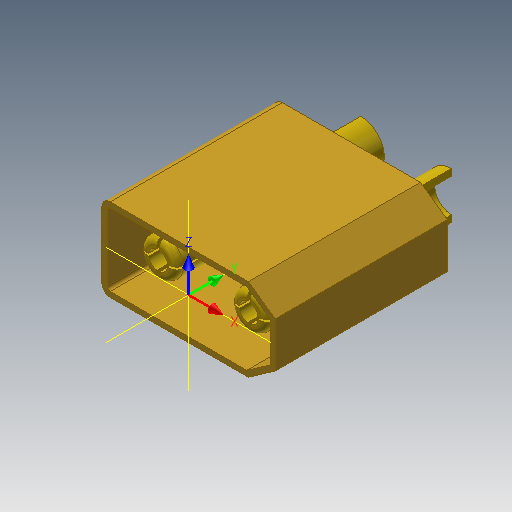
# Autodesk Inventor part: XT90 Male
Saved by Autodesk Inventor 2018 (Build 220112000, 112)
## iProperties
Created: 2021-08-31
Part Number: XT90 Male
Material: PPS-Kunststoff
Document SubType Name: Modeling
Designer: A. Gieck
Mass: 3.12149 g
Surface Area: 36.0039 cm^2
Volume: 1.90683 cm^3
Density: 1.637 g/cm^3
Appearance: Stecker Orange
RuleStatus: InUse
Author: A. Gieck
Autodesk Inventor part; units mm, degrees
ref_plane "YZ Plane" through (0, 0, 0) normal (1, 0, 0) x (0, 1, 0)
ref_plane "XZ Plane" through (0, 0, 0) normal (0, 1, 0) x (-1, 0, 0)
ref_plane "XY Plane" through (0, 0, 0) normal (0, 0, 1) x (1, 0, 0)
sketch "Skizze5" plane through (0, 0, 0) normal (0, 1, 0) x (-1, 0, 0)
  line L0 (10.475, 5) -> (-10.475, 5) construction
  line L1 (-10.475, 5) -> (-10.475, -5) construction
  line L2 (-10.475, -5) -> (10.475, -5) construction
  line L3 (10.475, -5) -> (10.475, 5) construction
  line L4 (9.475, 5) -> (-7.226, 5)
  line L5 (-7.226, 5) -> (-7.226, -5) construction
  line L6 (-7.226, -5) -> (9.475, -5)
  line L7 (10.475, -4) -> (10.475, 4)
  line L8 (-7.226, -5) -> (-10.475, -2.725)
  line L9 (-10.475, -2.725) -> (-10.475, 2.725)
  line L10 (-7.226, 5) -> (-10.475, 2.725)
  arc A0 (10.475, 4) -> (9.475, 5) centre (9.475, 4) ccw
  arc A1 (9.475, -5) -> (10.475, -4) centre (9.475, -4) ccw
  line L11 (-7.0305, 4.38) -> (9.475, 4.38)
  arc A2 (9.855, 4) -> (9.475, 4.38) centre (9.475, 4) ccw
  line L12 (9.855, 4) -> (9.855, -4)
  arc A3 (9.475, -4.38) -> (9.855, -4) centre (9.475, -4) ccw
  line L13 (9.475, -4.38) -> (-7.0305, -4.38)
  line L14 (-7.0305, -4.38) -> (-9.855, -2.4022)
  line L15 (-9.855, -2.4022) -> (-9.855, 2.4022)
  line L16 (-9.855, 2.4022) -> (-7.0305, 4.38)
  circle A4 centre (5.475, 0) radius 2.25
  circle A5 centre (-5.475, 0) radius 2.25
  line L17 (5.475, 0) -> (-5.475, 0) construction
  point P0 (0, 0)
  point P1 (-10.475, 0)
  point P2 (-10.475, 0)
  point P3 (0, 5)
  point P4 (0, 0)
  dimension "d40" = 20.95
  dimension "d41" = 10
  dimension "d42" = 5.45
  dimension "d43" = 55
  dimension "d44" = 17.701
  dimension "d45" = 1
  dimension "d46" = 0.62
  dimension "d47" = 10.95
  dimension "d48" = 4.5
  constraints: 36 end point, 8 point on circle, 6 centre point, 5 parallel, 5 point on line, 4 midpoint, 4 tangent, 3 horizontal, 2 coincident, 2 equal radius, 2 perpendicular, 1 horizontal alignment, 1 vertical alignment, 7 other
  measures "d40" distance of L0.start L0.end
  measures "d41" distance of L0.end L1.end
  measures "d42" distance of L8.end L9.end
  measures "d43" angle of L1 L10
  measures "d44" distance of L0.start L4.end
  measures "d45" radius of A0
  measures "d46" distance between parallel lines of L4 L11
  measures "d47" distance of L17.end L17.start
  measures "d48" diameter of A4
extrude "Extrusion1" add sketch "Skizze5" along normal blind 14
sketch "Skizze6" plane through (0, 14, 0) normal (0, 1, 0) x (1, 0, 0)
  arc A0 (-9.855, -4) -> (-9.475, -4.38) centre (-9.475, -4) ccw projected
  line L0 (-9.855, -4) -> (-9.855, 4) construction
  arc A1 (-9.475, 4.38) -> (-9.855, 4) centre (-9.475, 4) ccw construction
  line L1 (-9.475, 4.38) -> (7.0305, 4.38) construction
  line L2 (7.0305, 4.38) -> (9.855, 2.4022) construction
  line L3 (9.855, 2.4022) -> (9.855, -2.4022) construction
  line L4 (9.855, -2.4022) -> (7.0305, -4.38) construction
  line L5 (7.0305, -4.38) -> (-9.475, -4.38) construction
  line L6 (7.226, 5) -> (-9.475, 5) projected
  arc A2 (-9.475, 5) -> (-10.475, 4) centre (-9.475, 4) ccw projected
  line L7 (-10.475, 4) -> (-10.475, -4) projected
  arc A3 (-10.475, -4) -> (-9.475, -5) centre (-9.475, -4) ccw projected
  line L8 (-9.475, -5) -> (7.226, -5) projected
  line L9 (7.226, -5) -> (10.475, -2.725) projected
  line L10 (10.475, -2.725) -> (10.475, 2.725) projected
  line L11 (10.475, 2.725) -> (7.226, 5) projected
  point P0 (0, 0)
extrude "Extrusion2" add sketch "Skizze6" along normal blind 6.8
sketch "Skizze7" plane through (-5.475, 0, 0) normal (0, -1, 0) x (1, 0, 0)
  circle A0 centre (0, 0) radius 2.25 projected
  circle A1 centre (10.95, 0) radius 2.25 projected
  point P0 (5.475, 0)
extrude "Extrusion3" cut sketch "Skizze7" against normal blind 1.8
sketch "Skizze8" plane through (0, 20.8, 0) normal (0, 1, 0) x (1, 0, 0)
  circle A0 centre (-5.475, 0) radius 2.25 construction
  circle A1 centre (5.475, 0) radius 2.25 construction
  circle A2 centre (-5.475, 0) radius 2.825
  circle A3 centre (5.475, 0) radius 2.825
  circle A4 centre (-5.475, 0) radius 2.025
  circle A5 centre (5.475, 0) radius 2.025
  point P0 (0, 0)
  dimension "d55" = 5.65
  dimension "d56" = 4.05
  constraints: 4 centre point, 4 coincident, 2 equal radius
  measures "d55" diameter of A2
  measures "d56" diameter of A4
extrude "Extrusion4" add sketch "Skizze8" along normal blind 5.5
sketch "Skizze9" plane through (-5.475, 26.3, 0) normal (0, 1, 0) x (1, 0, 0)
  circle A0 centre (0, 0) radius 2.025 projected
  circle A1 centre (0, 0) radius 2.825 projected
  circle A2 centre (10.95, 0) radius 2.025 projected
  circle A3 centre (10.95, 0) radius 2.825 projected
  line L0 (0, 2.825) -> (0, -2.825)
  line L1 (10.95, 2.825) -> (10.95, -2.825)
  point P0 (5.475, 0)
  constraints: 4 end point, 4 point on circle, 1 parallel, 1 vertical
extrude "Extrusion5" cut sketch "Skizze9" against normal blind 4.6 contours L0 A0 | A0 L0 A1 | A2 L1 | A2 L1 A3 picked at (-0.6311, -0.2394) picked at (-2.5397, 0.0814) picked at (11.2429, 0.6082) picked at (13.4678, -0.3597)
sketch "Skizze10" plane through (0, 20.8, 0) normal (0, 1, 0) x (1, 0, 0)
  circle A0 centre (-5.475, 0) radius 2.825 projected
  circle A1 centre (5.475, 0) radius 2.825 projected
  circle A2 centre (-5.475, 0) radius 4.2
  circle A3 centre (5.475, 0) radius 4.2
  circle A4 centre (-5.475, 0) radius 2.025 projected
  circle A5 centre (5.475, 0) radius 2.025 projected
  point P0 (0, 0)
  dimension "d61" = 8.4
  constraints: 2 centre point, 2 coincident, 1 equal radius
  measures "d61" diameter of A2
extrude "Extrusion6" cut sketch "Skizze10" against normal blind 3
sketch "Skizze11" plane through (-5.475, 1.8, 0) normal (0, -1, 0) x (1, 0, 0)
  circle A0 centre (0, 0) radius 2.25 projected
  circle A1 centre (10.95, 0) radius 2.25 projected
  line L0 (-2.25, 0.15) -> (2.25, 0.15)
  line L1 (2.25, 0.15) -> (2.25, -0.15)
  line L2 (2.25, -0.15) -> (-2.25, -0.15)
  line L3 (-2.25, -0.15) -> (-2.25, 0.15)
  line L4 (-0.15, 2.25) -> (0.15, 2.25)
  line L5 (0.15, 2.25) -> (0.15, -2.25)
  line L6 (0.15, -2.25) -> (-0.15, -2.25)
  line L7 (-0.15, -2.25) -> (-0.15, 2.25)
  line L8 (8.7, 0.15) -> (13.2, 0.15)
  line L9 (13.2, 0.15) -> (13.2, -0.15)
  line L10 (13.2, -0.15) -> (8.7, -0.15)
  line L11 (8.7, -0.15) -> (8.7, 0.15)
  line L12 (10.8, 2.25) -> (11.1, 2.25)
  line L13 (11.1, 2.25) -> (11.1, -2.25)
  line L14 (11.1, -2.25) -> (10.8, -2.25)
  line L15 (10.8, -2.25) -> (10.8, 2.25)
  circle A2 centre (0, 0) radius 1.15
  circle A3 centre (10.95, 0) radius 1.15
  point P0 (5.475, 0)
  point P1 (0, 2.25)
  point P2 (10.95, 2.25)
  point P3 (-2.25, 0)
  point P4 (8.7, 0)
  dimension "d64" = 0.3
  dimension "d68" = 2.3
  constraints: 32 end point, 8 parallel, 8 tangent, 7 perpendicular, 4 horizontal, 4 midpoint, 2 centre point, 2 coincident, 2 horizontal alignment, 2 vertical alignment, 1 equal radius
  measures "d64" distance of L0.end L1.end
  measures "d68" diameter of A2
fillet "Rundung2" radius 0.8 2 edges at (-3.225, 1.8, 0) (7.725, 1.8, 0)
extrude "Extrusion7" cut sketch "Skizze11" against normal up to surface (12.2 mm away) contours A0 L2 A2 L0 | L1 L2 A0 | A0 L0 L1 | L5 A2 L7 A0 | A0 L4 L5 | A2 L2 L5 L0 | L0 L5 A2 | L5 L6 A0 | A0 L7 A2 L5 | A2 L5 L2 | A0 L7 L4 | L5 L0 L7 A2 | L5 L2 L7 L0 | L6 L7 A0 | A2 L7 L2 L5 | L7 L0 A2 | L7 L2 A2 L0 | A2 L2 L7 | L0 A2 L2 A0 | A0 L3 L0 | L2 L3 A0 | A1 L10 A3 L8 | L9 L10 A1 | A1 L8 L9 | L13 A3 L15 A1 | A1 L12 L13 | A3 L10 L13 L8 | L8 L13 A3 | L13 L14 A1 | A1 L15 A3 L13 | A3 L13 L10 | A1 L15 L12 | L13 L8 L15 A3 | L13 L10 L15 L8 | L14 L15 A1 | A3 L15 L10 L13 | L15 L8 A3 | L15 L10 A3 L8 | A3 L10 L15 | L8 A3 L10 A1 | A1 L11 L8 | L10 L11 A1
sketch "Skizze12" plane through (5.475, 17.8, 0) normal (0, 1, 0) x (1, 0, 0)
  circle A0 centre (0, 0) radius 2.025 projected
  circle A1 centre (-10.95, 0) radius 2.025 projected
  point P0 (-5.475, 0)
extrude "Extrusion8" cut sketch "Skizze12" against normal blind 3
chamfer "Fase1" distance 2 angle 45 2 edges at (3.45, 14.8, 0) (-7.5, 14.8, 0)
sketch "Skizze13" plane through (0, 14, 0) normal (0, -1, 0) x (1, 0, 0)
  circle A0 centre (5.475, 0) radius 2.825 projected
  circle A1 centre (-5.475, 0) radius 2.825 projected
  point P0 (0, 0)
extrude "Extrusion9" add sketch "Skizze13" along normal blind 0.8
